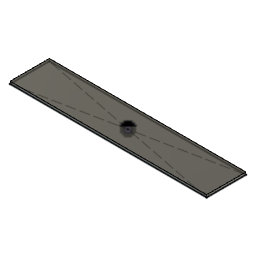
Assembly_box v7 (Autodesk Fusion 360 archive; units mm, degrees)
design "length"
Autodesk Fusion 360 part; units mm, degrees
sketch "Sketch1" plane through (0, 0, 0) normal (0, 0, 1) x (1, 0, 0)
  line L0 (125, -25) -> (-125, -25)
  line L1 (-125, -25) -> (-125, 25)
  line L2 (-125, 25) -> (125, 25)
  line L3 (125, 25) -> (125, -25)
  line L4 (125, -25) -> (-125, 25) construction
  line L5 (-125, -25) -> (125, 25) construction
  dimension "d1" = 250
  dimension "d2" = 50
  constraint horizontal L0
  constraint perpendicular L0 L1
  constraint parallel L0 L2
  constraint parallel L1 L3
  constraint coincident L4 origin
  constraint coincident L5 origin
extrude "Extrude1" add sketch "Sketch1" along normal blind 3

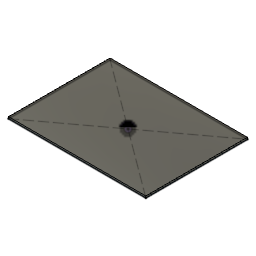
design "buttom"
Autodesk Fusion 360 part; units mm, degrees
sketch "Sketch1" plane through (0, 0, 0) normal (0, 0, 1) x (1, 0, 0)
  line L0 (125, -92.5) -> (-125, -92.5)
  line L1 (-125, -92.5) -> (-125, 92.5)
  line L2 (-125, 92.5) -> (125, 92.5)
  line L3 (125, 92.5) -> (125, -92.5)
  line L4 (125, -92.5) -> (-125, 92.5) construction
  line L5 (-125, -92.5) -> (125, 92.5) construction
  dimension "d1" = 250
  dimension "d2" = 185
  constraint horizontal L0
  constraint perpendicular L0 L1
  constraint parallel L0 L2
  constraint parallel L1 L3
  constraint coincident L4 origin
  constraint coincident L5 origin
  measures "d1" distance of L1.end L2.end
  measures "d2" distance of L0.end L1.end
extrude "Extrude1" add sketch "Sketch1" along normal blind 3

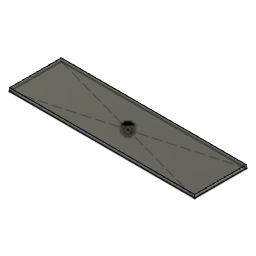
design "width"
Autodesk Fusion 360 part; units mm, degrees
sketch "Sketch1" plane through (0, 0, 0) normal (0, 0, 1) x (1, 0, 0)
  line L0 (89.5, -25) -> (-89.5, -25)
  line L1 (-89.5, -25) -> (-89.5, 25)
  line L2 (-89.5, 25) -> (89.5, 25)
  line L3 (89.5, 25) -> (89.5, -25)
  line L4 (89.5, -25) -> (-89.5, 25) construction
  line L5 (-89.5, -25) -> (89.5, 25) construction
  dimension "d1" = 179
  dimension "d2" = 50
  constraint horizontal L0
  constraint perpendicular L0 L1
  constraint parallel L0 L2
  constraint parallel L1 L3
  constraint coincident L4 origin
  constraint coincident L5 origin
  measures "d1" distance of L1.end L2.end
  measures "d2" distance of L0.end L1.end
extrude "Extrude1" add sketch "Sketch1" along normal blind 3
ref_plane "WorkPlane1" through (0, 0, 3) normal (0, 0, 1) x (1, 0, 0)
sketch "Sketch2" plane through (0, 0, 3) normal (0, 0, 1) x (1, 0, 0)
